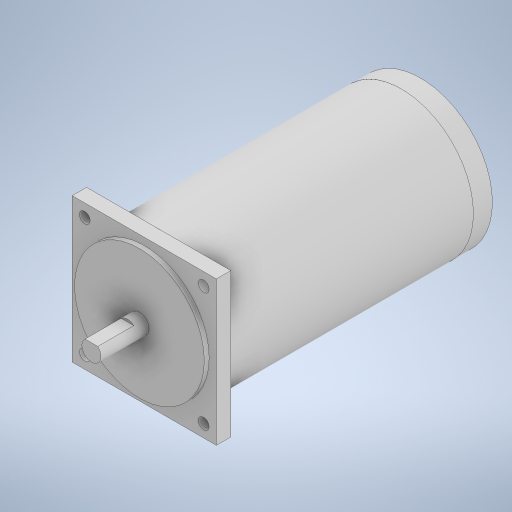
# Autodesk Inventor part: 중형 모터 MB60080-2430 DC24V
Saved by Autodesk Inventor 2023 (Build 270158000, 158)
## iProperties
Created: 2022-06-19
Part Number: 중형 모터 MB60080-2430 DC24V
Material: 일반
Document SubType Name: Modeling
Designer: fly01
Density: 1 g/cm^3
Appearance: 기본값
Author: fly01
Autodesk Inventor part; units mm, degrees
ref_plane "YZ Plane" through (0, 0, 0) normal (1, 0, 0) x (0, 1, 0)
ref_plane "XZ Plane" through (0, 0, 0) normal (0, 1, 0) x (-1, 0, 0)
ref_plane "XY Plane" through (0, 0, 0) normal (0, 0, 1) x (1, 0, 0)
sketch "스케치1" plane through (0, 0, 0) normal (0, 0, 1) x (1, 0, 0)
  line L0 (-30, -30) -> (30, -30)
  line L1 (30, -30) -> (30, 30)
  line L2 (30, 30) -> (-30, 30)
  line L3 (-30, 30) -> (-30, -30)
  line L4 (-30, -30) -> (30, 30) construction
  line L5 (30, -30) -> (-30, 30) construction
  circle A0 centre (0, 0) radius 30
  circle A1 centre (-24.7487, 24.7487) radius 2.25
  circle A2 centre (0, 0) radius 35 construction
  circle A3 centre (-24.7487, -24.7487) radius 2.25
  circle A4 centre (24.7487, -24.7487) radius 2.25
  circle A5 centre (24.7487, 24.7487) radius 2.25
  dimension "d3" = 70
  dimension "d0" = 60
  dimension "d1" = 60
  dimension "d2" = 4.5
  dimension "d6" = 360
  constraints: 12 end point, 5 centre point, 2 coincident, 2 midpoint, 2 parallel, 1 horizontal, 1 perpendicular, 1 point on line, 12 other
  measures "d0" distance of L2.end L1.end
  measures "d1" distance of L1.end L0.end
  measures "d2" diameter of A1
extrude "돌출1" add sketch "스케치1" along normal blind 6
extrude "돌출2" add sketch "스케치1" against normal blind 109 contours A0
sketch "스케치2" plane through (0, 0, -109) normal (0, 0, -1) x (-1, 0, 0)
  circle A0 centre (0, 0) radius 30 projected
  circle A1 centre (0, 0) radius 29.9
  dimension "d12" = 0.1
  constraints: 1 centre point
  measures "d12" radial gap between concentric circles of A0 A1
extrude "돌출3" cut sketch "스케치2" against normal blind 8
sketch "스케치3" plane through (0, 0, 6) normal (0, 0, 1) x (1, 0, 0)
  circle A0 centre (0, 0) radius 27
  dimension "d15" = 54
  constraints: 1 centre point, 1 coincident
  measures "d15" diameter of A0
extrude "돌출4" add sketch "스케치3" along normal blind 2
sketch "스케치4" plane through (0, 0, 8) normal (0, 0, 1) x (1, 0, 0)
  circle A0 centre (0, 0) radius 4
  line L0 (-2.6458, 3) -> (2.6458, 3)
  line L1 (0, 3) -> (0, -4)
  dimension "d18" = 8
  dimension "d19" = 7
  constraints: 4 end point, 3 point on circle, 1 centre point, 1 coincident, 1 horizontal, 1 midpoint
  measures "d18" diameter of A0
  measures "d19" distance of L1.start L1.end
extrude "돌출5" add sketch "스케치4" along normal blind 20 contours A0 L1 L0 | A0 L0 L1
extrude "돌출6" add sketch "스케치4" along normal blind 5 contours L0 A0
